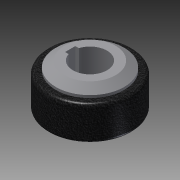
# Autodesk Inventor part: 砂轮
Saved by Autodesk Inventor 2015 (Build 190159000, 159)
## iProperties
Created: 2017-05-11
Part Number: 砂轮
Material: 常规
Document SubType Name: Modeling
Designer: Administrator
Density: 1 g/cm^3
Appearance: 默认
Author: Administrator
Autodesk Inventor part; units mm, degrees
ref_plane "YZ Plane" through (0, 0, 0) normal (1, 0, 0) x (0, 1, 0)
ref_plane "XZ Plane" through (0, 0, 0) normal (0, 1, 0) x (-1, 0, 0)
ref_plane "XY Plane" through (0, 0, 0) normal (0, 0, 1) x (1, 0, 0)
sketch "草图1" plane through (0, 0, 0) normal (0, 0, 1) x (1, 0, 0)
  circle A0 centre (0, 0) radius 24.5
  dimension "d0" = 49
  constraints: 1 centre point, 1 coincident
  measures "d0" diameter of A0
extrude "拉伸1" add sketch "草图1" along normal blind 20
sketch "草图2" plane through (0, 0, 20) normal (0, 0, 1) x (1, 0, 0)
  circle A0 centre (0, 0) radius 20
  dimension "d3" = 40
  constraints: 1 centre point, 1 coincident
  measures "d3" diameter of A0
extrude "拉伸2" add sketch "草图2" along normal blind 5
chamfer "倒角1" distance 5 distance2 3.5 1 edges at (-20, 0, 25) measured on face at (-2.364, 6.2334, 25)
sketch "草图3" plane through (0, 0, 0) normal (0, 0, -1) x (-1, 0, 0)
  circle A0 centre (0, 0) radius 20
  dimension "d9" = 40
  constraints: 1 centre point, 1 coincident
  measures "d9" diameter of A0
extrude "拉伸3" add sketch "草图3" along normal blind 5
chamfer "倒角2" distance 5 distance2 3.5 1 edges at (20, 0, -5) measured on face at (-7.896, -2.3423, -5)
fillet "圆角1" radius 2 2 edges at (-24.5, 0, 0) (-24.5, 0, 20)
sketch "草图4" plane through (0, 0, -5) normal (0, 0, -1) x (-1, 0, 0)
  circle A0 centre (0, 0) radius 10
  line L0 (11.6, 3) -> (9.5394, 3)
  line L1 (9.5394, 3) -> (9.5394, -3)
  line L2 (9.5394, -3) -> (11.6, -3)
  line L3 (11.6, -3) -> (11.6, 3)
  dimension "d16" = 20
  dimension "d17" = 6
  dimension "d18" = 11.6
  constraints: 8 end point, 2 parallel, 2 point on circle, 1 centre point, 1 coincident, 1 horizontal, 1 perpendicular
  measures "d16" diameter of A0
  measures "d17" distance of L2.end L0.start
  measures "d18" distance from line of point (0, 0) L3
extrude "拉伸4" cut sketch "草图4" against normal through all
